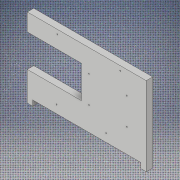
# Autodesk Inventor part: cerceau_front
Saved by Autodesk Inventor 2019 (Build 230136000, 136)
## iProperties
Created: 2019-05-16
Part Number: cerceau_front
Material: Générique
Document SubType Name: Modeling
Designer: thoma
Density: 1 g/cm^3
Appearance: Par défaut
Author: thoma
Autodesk Inventor part; units mm, degrees
ref_plane "YZ Plane" through (0, 0, 0) normal (1, 0, 0) x (0, 1, 0)
ref_plane "XZ Plane" through (0, 0, 0) normal (0, 1, 0) x (-1, 0, 0)
ref_plane "XY Plane" through (0, 0, 0) normal (0, 0, 1) x (1, 0, 0)
sketch "Sketch1" plane through (0, 0, 0) normal (0, 0, 1) x (1, 0, 0)
  line L0 (0, 0) -> (110, 0)
  line L1 (110, 0) -> (110, 73)
  line L2 (110, 73) -> (0, 73)
  line L3 (6, 57) -> (50, 57)
  line L4 (50, 57) -> (50, 27)
  line L5 (6, 57) -> (0, 57)
  line L6 (0, 73) -> (0, 57)
  line L7 (0, 27) -> (0, 0)
  line L8 (0, 27) -> (50, 27)
  dimension "d0" = 110
  dimension "d2" = 16
  dimension "d19" = 57
  dimension "d22" = 50
  dimension "d66" = 30
  constraints: 18 end point, 3 horizontal, 3 parallel, 1 perpendicular
  measures "d0" distance of L2.end L1.end
  measures "d2" distance between parallel lines of L2 L3
  measures "d19" distance between parallel lines of L0 L3
  measures "d22" distance of L7.start L4.end
  measures "d66" distance of L3.end L4.end
extrude "Extrusion1" add sketch "Sketch1" along normal blind 6
sketch "Sketch2" plane through (0, 0, 6) normal (0, 0, 1) x (1, 0, 0)
  line L0 (105, 0) -> (105, 5)
  line L1 (105, 5) -> (5, 5)
  line L2 (5, 5) -> (5, 0)
  line L3 (0, 27) -> (0, 0) projected
  line L4 (0, 0) -> (110, 0) projected
  dimension "d13" = 100
  dimension "d14" = 5
  dimension "d15" = 5
  constraints: 6 end point, 1 parallel
  measures "d13" distance of L0.end L1.end
  measures "d14" distance between parallel lines of L3 L2
  measures "d15" distance between parallel lines of L4 L1
extrude "Extrusion2" cut sketch "Sketch2" against normal blind 10
sketch "Sketch3" plane through (0, 0, 0) normal (0, 0, -1) x (-1, 0, 0)
  line L0 (-331.8351, -68) -> (-331.8351, 72) construction
  line L1 (218.6881, -67.4159) -> (-331.3119, -67.4159)
  line L2 (-331.8351, 72) -> (218.1649, 72)
  line L3 (-50.021, 72.5841) -> (-50.021, -67.4159)
  line L4 (-301.8351, 60.0199) -> (-301.8351, -95.3329) construction
  line L5 (-194.8351, 50.8275) -> (-194.8351, -92.5752) construction
  line L6 (-289.8351, 60.0199) -> (-289.8351, -99.0099) construction
  line L7 (-182.8351, -92.5752) -> (-182.8351, 81.6223) construction
  line L8 (-224.6619, -78.1083) -> (-224.6619, -12.2159) construction
  line L9 (-184.2519, -76.0321) -> (-184.2519, -10.2421) construction
  line L10 (-223.8335, -61.4159) -> (-147.922, -61.4159) construction
  line L11 (-179.8519, -67.4159) -> (-179.8519, -42.4159) construction
  line L12 (-229.1619, -42.4159) -> (-229.1619, -67.4159) construction
  line L13 (-73.021, 109.947) -> (-73.021, -118.6448) construction
  line L14 (-147.521, 95.654) -> (-147.521, -118.6448) construction
  line L15 (-208.521, 101.2387) -> (-208.521, -106.3335) construction
  line L16 (-237.7385, -71.614) -> (-237.7385, -46.614)
  line L17 (243.9615, -46.614) -> (243.9615, -71.614)
  line L18 (-92.021, 52) -> (-57.021, 52) construction
  line L19 (-57.021, 52) -> (-57.021, 27) construction
  line L20 (-57.021, 27) -> (-92.021, 27) construction
  line L21 (-92.021, 27) -> (-92.021, 52) construction
  line L22 (-301.8351, 2.5165) -> (201.7932, 2.5165) construction
  line L23 (-105, 0) -> (-105, 5) projected
  line L24 (-105, 5) -> (-5, 5) projected
  line L25 (-5, 5) -> (-5, 0) projected
  line L26 (0, 0) -> (-5, 0) projected
  line L27 (0, 27) -> (0, 0) projected
  line L28 (-50, 27) -> (0, 27) projected
  line L29 (-50, 57) -> (-50, 27) projected
  line L30 (0, 57) -> (-50, 57) projected
  line L31 (0, 73) -> (0, 57) projected
  line L32 (-110, 73) -> (0, 73) projected
  line L33 (-110, 0) -> (-110, 73) projected
  line L34 (-105, 0) -> (-110, 0) projected
  point P0 (-53.9258, 1.4801)
  point P1 (-331.3119, -67.4159)
  point P2 (-266.7948, -13.3199)
  point P3 (-301.8351, 60.0199)
  point P4 (-301.8351, -95.3329)
  point P5 (-289.8351, 2.5165)
  point P6 (-194.8351, 2.5165)
  point P7 (-182.8351, 2.5165)
  point P8 (189.7932, 2.5165)
  point P9 (94.7932, 2.5165)
  point P10 (82.7932, 2.5165)
  point P11 (-50.021, -58.9159)
  point P12 (-224.6619, -61.4159)
  point P13 (-184.2519, -61.4159)
  point P14 (124.6199, -61.4159)
  point P15 (84.2099, -61.4159)
  point P16 (-73.021, 12.3841)
  point P17 (-27.021, 12.3841)
  point P18 (-319.3351, 69)
  point P19 (-261.0351, 69)
  point P20 (-202.7351, 69)
  point P21 (-144.4351, 69)
  point P22 (-86.1351, 69)
  point P23 (-27.8351, 69)
  point P24 (30.4649, 69)
  point P25 (88.7649, 69)
  point P26 (147.0649, 69)
  point P27 (205.3649, 69)
  point P28 (-325.3351, 62)
  point P29 (-325.3351, 54)
  point P30 (-325.3351, 46)
  point P31 (-325.3351, 38)
  point P32 (-325.3351, 30)
  point P33 (-325.3351, 22)
  point P34 (-325.3351, 14)
  point P35 (-325.3351, 6)
  point P36 (-325.3351, -2)
  point P37 (-325.3351, -10)
  point P38 (-325.3351, -18)
  point P39 (-325.3351, -26)
  point P40 (-325.3351, -34)
  point P41 (225.2932, -34)
  point P42 (225.2932, -26)
  point P43 (225.2932, -18)
  point P44 (225.2932, -10)
  point P45 (225.2932, -2)
  point P46 (225.2932, 6)
  point P47 (225.2932, 14)
  point P48 (225.2932, 22)
  point P49 (225.2932, 30)
  point P50 (225.2932, 38)
  point P51 (225.2932, 46)
  point P52 (225.2932, 54)
  point P53 (225.2932, 62)
  point P54 (-242.2385, -65.614)
  point P55 (248.4615, -65.614)
  dimension "d32" = 30
  dimension "d33" = 12
  dimension "d34" = 137
  dimension "d35" = 12
  dimension "d36" = 8.5
  dimension "d37" = 4.4
  dimension "d38" = 4.5
  dimension "d39" = 6
  dimension "d40" = 23
  dimension "d41" = 97.5
  dimension "d42" = 158.5
  dimension "d43" = 3
  dimension "d44" = 12.5
  dimension "d45" = 58.3
  dimension "d46" = 6.5
  dimension "d47" = 10
  dimension "d48" = 8
  dimension "d49" = 35
  dimension "d50" = 35
  dimension "d51" = 25
  dimension "d52" = 4.5
  dimension "d53" = 4.5
  dimension "d56" = 20
  dimension "d57" = 7
  dimension "d58" = 1
  constraints: 36 end point, 29 horizontal alignment, 12 vertical alignment, 11 point on line, 8 vertical, 3 perpendicular, 2 horizontal, 17 other
  measures "d35" distance between parallel lines of L5 L7
  measures "d37" distance between parallel lines of L9 L11
  measures "d38" distance between parallel lines of L12 L8
  measures "d45" distance of point (-319.335, 69) point (-261.035, 69)
  measures "d48" distance of point (-325.335, 62) point (-325.335, 54)
  measures "d49" distance of L18.end L18.start
  measures "d50" distance of L20.end L19.end
  measures "d51" distance of L20.end L18.start
  measures "d52" distance from line of L16 point (-242.238, -65.614)
  measures "d53" distance from line of L17 point (248.462, -65.614)
hole "Hole1" at (50.021, -58.9159, 0) at (301.8351, 2.5165, 0) at (242.2385, -65.614, 0) at (194.8351, 2.5165, 0) at (289.8351, 2.5165, 0) at (182.8351, 2.5165, 0) at (-189.7932, 2.5165, 0) at (-201.7932, 2.5165, 0) at (-94.7932, 2.5165, 0) at (-82.7932, 2.5165, 0) at (224.6619, -61.4159, 0) at (184.2519, -61.4159, 0) at (-124.6199, -61.4159, 0) at (-84.2099, -61.4159, 0) at (73.021, 12.3841, 0) at (27.021, 12.3841, 0) at (325.3351, 62, 0) at (325.3351, 54, 0) at (325.3351, 46, 0) at (325.3351, 38, 0) at (325.3351, 30, 0) at (325.3351, 22, 0) at (325.3351, 14, 0) at (325.3351, 6, 0) at (325.3351, -2, 0) at (325.3351, -10, 0) at (325.3351, -18, 0) at (325.3351, -26, 0) at (325.3351, -34, 0) at (-225.2932, -34, 0) at (-225.2932, -26, 0) at (-225.2932, -18, 0) at (-225.2932, -10, 0) at (-225.2932, -2, 0) at (-225.2932, 6, 0) at (-225.2932, 14, 0) at (-225.2932, 22, 0) at (-225.2932, 30, 0) at (-225.2932, 38, 0) at (-225.2932, 46, 0) at (-225.2932, 54, 0) at (-225.2932, 62, 0) at (57.021, 52, 0) at (57.021, 27, 0) at (92.021, 27, 0) at (92.021, 52, 0) at (-248.4615, -65.614, 0) at (27.8351, 69, 0) at (86.1351, 69, 0) direction (0, 0, 1) diameter 1 end through all
body "Solid1"
